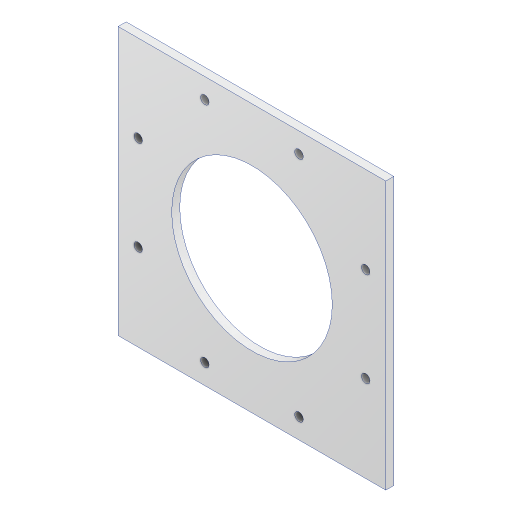
# Autodesk Inventor part: base_plate
Saved by Autodesk Inventor 2024.3 (Build 283343000, 343)
## iProperties
Created: 2024-10-12
Part Number: base_plate
Material: アルミニウム 6061
Document SubType Name: Modeling
Designer: haya
Density: 2.7 g/cm^3
Appearance: アルミニウム - フラット
Mass: 40.5 g
Surface Area: 206 cm^2
Volume: 15 cm^3
Author: haya
Autodesk Inventor part; units mm, degrees
ref_plane "YZ Plane" through (0, 0, 0) normal (1, 0, 0) x (0, 1, 0)
ref_plane "XZ Plane" through (0, 0, 0) normal (0, 1, 0) x (-1, 0, 0)
ref_plane "XY Plane" through (0, 0, 0) normal (0, 0, 1) x (1, 0, 0)
sketch "スケッチ1" plane through (0, 0, 0) normal (0, 0, 1) x (1, 0, 0)
  line L0 (-50, 50) -> (50, 50)
  line L1 (50, 50) -> (50, -50)
  line L2 (50, -50) -> (-50, -50)
  line L3 (-50, -50) -> (-50, 50)
  line L4 (0, 0) -> (0, 50) construction
  line L5 (0, 0) -> (50, 0) construction
  dimension "d0" = 100
  dimension "d1" = 100
  constraints: 12 end point, 3 perpendicular, 2 midpoint, 2 parallel, 1 horizontal, 2 other
  measures "d0" distance of L0.start L0.end
  measures "d1" distance of L0.end L1.end
extrude "押し出し1" add sketch "スケッチ1" along normal blind 3
sketch "スケッチ2" plane through (0, 0, 3) normal (0, 0, 1) x (1, 0, 0)
  point P0 (0, 0)
  point P1 (0, 0)
  constraints: 1 coincident
hole "穴1" at (0, 0, 3) direction (0, 0, -1) diameter 60 end through all
sketch "スケッチ3" plane through (0, 0, 3) normal (0, 0, 1) x (1, 0, 0)
  line L0 (0, 0) -> (0, 50) construction
  line L1 (50, 50) -> (-50, 50) projected
  line L2 (0, 0) -> (19.8012, 47.8043) construction
  point P0 (17.6034, 42.4985)
  point P1 (-17.6034, 42.4985)
  point P2 (-42.4985, 17.6034)
  point P3 (-42.4985, -17.6034)
  point P4 (-17.6034, -42.4985)
  point P5 (17.6034, -42.4985)
  point P6 (42.4985, -17.6034)
  point P7 (42.4985, 17.6034)
  dimension "d11" = 22.5
  dimension "d12" = 46
  dimension "d15" = 360
  constraints: 4 end point, 1 midpoint, 1 point on line, 9 other
  measures "d11" angle of L0 L2
  measures "d12" distance of point (17.603, 42.498) L0.start
hole "穴2" at (17.6034, 42.4985, 3) at (-17.6034, 42.4985, 3) at (-42.4985, 17.6034, 3) at (-42.4985, -17.6034, 3) at (-17.6034, -42.4985, 3) at (17.6034, -42.4985, 3) at (42.4985, -17.6034, 3) at (42.4985, 17.6034, 3) direction (0, 0, -1) diameter 3.2 end through all
